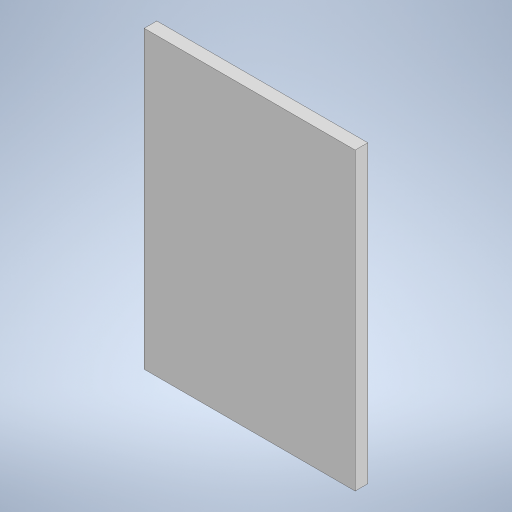
# Autodesk Inventor part: anushree frame
Saved by Autodesk Inventor 2023 (Build 270158000, 158)
## iProperties
Created: 2022-06-23
Part Number: anushree frame
Material: Generic
Document SubType Name: Modeling
Designer: ADITYA
Density: 1 g/cm^3
Appearance: Default
Author: ADITYA
Autodesk Inventor part; units mm, degrees
ref_plane "YZ Plane" through (0, 0, 0) normal (1, 0, 0) x (0, 1, 0)
ref_plane "XZ Plane" through (0, 0, 0) normal (0, 1, 0) x (-1, 0, 0)
ref_plane "XY Plane" through (0, 0, 0) normal (0, 0, 1) x (1, 0, 0)
sketch "Sketch1" plane through (0, 0, 0) normal (0, 0, 1) x (1, 0, 0)
  line L0 (-9.3024, 8.297) -> (240.6976, 8.297)
  line L1 (240.6976, 8.297) -> (240.6976, -341.703)
  line L2 (240.6976, -341.703) -> (-9.3024, -341.703)
  line L3 (-9.3024, -341.703) -> (-9.3024, 8.297)
  point P0 (0, 0)
  dimension "d0" = 250
  dimension "d1" = 350
  constraints: 8 end point, 2 parallel, 1 horizontal, 1 perpendicular
  measures "d0" distance of L1.end L2.end
  measures "d1" distance of L0.end L1.end
extrude "Extrusion1" add sketch "Sketch1" along normal blind 15
body "Solid1"
